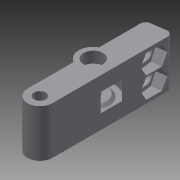
# Autodesk Inventor part: ExtruderSatoerBearingArm
Saved by Autodesk Inventor 2015 SP1 (Build 190203100, 203)
## iProperties
Created: 2015-05-02
Part Number: ExtruderSatoerBearingArm
Material: Generic
Document SubType Name: Modeling
Designer: Jack
Density: 1 g/cm^3
Appearance: Default
Author: Jack
Autodesk Inventor part; units mm, degrees
ref_plane "YZ Plane" through (0, 0, 0) normal (1, 0, 0) x (0, 1, 0)
ref_plane "XZ Plane" through (0, 0, 0) normal (0, 1, 0) x (-1, 0, 0)
ref_plane "XY Plane" through (0, 0, 0) normal (0, 0, 1) x (1, 0, 0)
sketch "Sketch1" plane through (0, 0, 0) normal (0, 0, 1) x (1, 0, 0)
  arc A0 (-4.75, 0) -> (4.75, 0) centre (0, 0) ccw
  line L0 (-4.75, 44.6649) -> (4.75, 46)
  line L1 (4.75, 46) -> (4.75, 0)
  arc A1 (-4.75, 27.0098) -> (-4.75, 17.7902) centre (-1.75, 22.4) ccw
  line L2 (-4.75, 0) -> (-4.75, 17.7902)
  line L3 (-4.75, 27.0098) -> (-4.75, 44.6649)
  dimension "d0" = 9.5
  dimension "d1" = 46
  dimension "d2" = 82
  dimension "d5" = 11
  dimension "d8" = 22.4
  dimension "d9" = 3
  constraints: 8 end point, 4 point on circle, 3 tangent, 3 vertical, 2 centre point, 1 coincident
  measures "d0" diameter of A0
  measures "d1" vertical distance of point (0, 0) L0.end
  measures "d2" angle of L1 L0
  measures "d5" diameter of A1
  measures "d8" vertical distance of point (0, 0) A1.centre
  measures "d9" distance from line of L3 A1.centre
extrude "Extrusion1" add sketch "Sketch1" along normal blind 18
sketch "Sketch4" plane through (0, 0, 18) normal (0, 0, 1) x (1, 0, 0)
  arc A0 (-4.75, 27.0098) -> (-4.75, 17.7902) centre (-1.75, 22.4) ccw projected
sketch "Sketch3" plane through (0, 0, 0) normal (0, 0, -1) x (-1, 0, 0)
  arc A0 (4.75, 17.7902) -> (4.75, 27.0098) centre (1.75, 22.4) ccw projected
  line L0 (1.75, 26.6724) -> (5.45, 24.5362)
  line L1 (5.45, 24.5362) -> (5.45, 20.2638)
  line L2 (5.45, 20.2638) -> (1.75, 18.1276)
  line L3 (1.75, 18.1276) -> (-1.95, 20.2638)
  line L4 (-1.95, 20.2638) -> (-1.95, 24.5362)
  line L5 (-1.95, 24.5362) -> (1.75, 26.6724)
  dimension "d17" = 7.4
  constraints: 12 end point, 1 coincident, 1 vertical, 13 other
  measures "d17" distance between parallel lines of L4 L1
extrude "Extrusion2" [suppressed]
hole "Hole2" at (-1.75, 22.4, 18) direction (0, 0, -1) diameter 4.5 end through all counterbore diameter 7.4 counterbore depth 4.2
ref_plane "Work Plane1" through (0, 0, 9) normal (0, 0, -1) x (-1, 0, 0)
sketch "Sketch5" plane through (0, 0, 9) normal (0, 0, -1) x (-1, 0, 0)
  arc A0 (-4.75, 0) -> (4.75, 0) centre (0, 0) ccw projected
  line L0 (4.75, 17.7902) -> (4.75, 0) projected
  arc A1 (4.75, 17.7902) -> (4.75, 27.0098) centre (1.75, 22.4) ccw projected
  line L1 (4.75, 44.6649) -> (4.75, 27.0098) projected
  line L2 (-4.75, 46) -> (4.75, 44.6649) projected
  line L3 (-4.75, 0) -> (-4.75, 46) projected
  circle A2 centre (1.75, 22.4) radius 8
  dimension "d28" = 16
  constraints: 1 centre point, 1 coincident
  measures "d28" diameter of A2
extrude "Extrusion3" [suppressed]
sketch "Sketch6" plane through (0, 0, 5.5) normal (0, 0, 1) x (1, 0, 0)
  circle A0 centre (-1.75, 22.4) radius 2.25 projected
  circle A1 centre (-1.75, 22.4) radius 5
  point P0 (0, 0)
  dimension "d31" = 10
  constraints: 1 centre point, 1 coincident
  measures "d31" diameter of A1
extrude "Extrusion4" [suppressed]
sketch "Sketch7" plane through (0, 0, 12.5) normal (0, 0, -1) x (-1, 0, 0)
  circle A0 centre (1.75, 22.4) radius 2.25 projected
  circle A1 centre (1.75, 22.4) radius 2.25 projected
  circle A2 centre (1.75, 22.4) radius 5 projected
  point P0 (0, 0)
extrude "Extrusion5" [suppressed]
chamfer "Chamfer1" [suppressed]
fillet "Fillet1" radius 2 2 edges at (-4.75, 44.6649, 9) (4.75, 46, 9)
sketch "Sketch8" plane through (-4.75, 29.8162, 5.5) normal (-1, 0, 0) x (0, 0, 1)
  line L0 (-5.5, 13.1101) -> (-5.5, -2.8064) projected
  line L1 (12.5, 13.1101) -> (12.5, -2.8064) projected
  line L2 (7.5, 7.9636) -> (7.5, 9.5636) construction
  line L3 (9.75, 7.9636) -> (9.75, 9.5636)
  line L4 (5.25, 9.5636) -> (5.25, 7.9636)
  arc A0 (5.25, 7.9636) -> (9.75, 7.9636) centre (7.5, 7.9636) ccw
  arc A1 (9.75, 9.5636) -> (5.25, 9.5636) centre (7.5, 9.5636) ccw
  line L5 (-5.5, 15.8636) -> (12.5, 15.8636) projected
  line L6 (-0.5, 7.9636) -> (-0.5, 9.5636) construction
  line L7 (1.75, 7.9636) -> (1.75, 9.5636)
  line L8 (-2.75, 9.5636) -> (-2.75, 7.9636)
  arc A2 (-2.75, 7.9636) -> (1.75, 7.9636) centre (-0.5, 7.9636) ccw
  arc A3 (1.75, 9.5636) -> (-2.75, 9.5636) centre (-0.5, 9.5636) ccw
  point P0 (-5.5, -29.8162)
  point P1 (7.5, 8.7636)
  point P2 (-0.5, 8.7636)
  dimension "d40" = 1.6
  dimension "d41" = 4.5
  dimension "d42" = 6.3
  dimension "d43" = 5
  dimension "d44" = 5
  constraints: 16 end point, 8 point on circle, 8 tangent, 4 centre point, 3 parallel, 2 midpoint, 2 vertical, 1 equal radius, 1 horizontal alignment
  measures "d40" distance of L2.start L2.end
  measures "d41" diameter of A1
  measures "d42" distance from line of L5 L2.end
  measures "d43" distance from line of L0 point (-0.5, 8.764)
  measures "d44" distance from line of L1 point (7.5, 8.764)
extrude "Extrusion6" cut sketch "Sketch8" against normal up to next
ref_plane "Work Plane2" through (4.75, 43.6993, 0) normal (0.9902681, 0.1391731, 0) x (0, 0, -1)
sketch "Sketch9" plane through (4.75, 43.6993, 0) normal (0.9902681, 0.1391731, 0) x (0, 0, -1)
  ellipse E0 centre (-5, -5.8619) end of major axis (-2.75, -5.8619) minor radius 2.2281 (-7.25, -5.8619) -> (-2.75, -5.8619) ccw projected
  ellipse E1 centre (-5, -4.2774) end of major axis (-7.25, -4.2774) minor radius 2.2281 (-2.75, -4.2774) -> (-7.25, -4.2774) ccw projected
  ellipse E2 centre (-13, -4.2774) end of major axis (-15.25, -4.2774) minor radius 2.2281 (-10.75, -4.2774) -> (-15.25, -4.2774) ccw projected
  ellipse E3 centre (-13, -5.8619) end of major axis (-10.75, -5.8619) minor radius 2.2281 (-15.25, -5.8619) -> (-10.75, -5.8619) ccw projected
  line L0 (-13, -10.1342) -> (-16.7, -7.9981)
  line L1 (-16.7, -7.9981) -> (-16.7, -3.7257)
  line L2 (-16.7, -3.7257) -> (-13, -1.5895)
  line L3 (-13, -1.5895) -> (-9.3, -3.7257)
  line L4 (-9.3, -3.7257) -> (-9.3, -7.9981)
  line L5 (-9.3, -7.9981) -> (-13, -10.1342)
  line L6 (-13, -0.005) -> (-9.3, -2.1412)
  line L7 (-9.3, -2.1412) -> (-9.3, -6.4136)
  line L8 (-9.3, -6.4136) -> (-13, -8.5498)
  line L9 (-13, -8.5498) -> (-16.7, -6.4136)
  line L10 (-16.7, -6.4136) -> (-16.7, -2.1412)
  line L11 (-16.7, -2.1412) -> (-13, -0.005)
  line L12 (-5, -10.1342) -> (-8.7, -7.9981)
  line L13 (-8.7, -7.9981) -> (-8.7, -3.7257)
  line L14 (-8.7, -3.7257) -> (-5, -1.5895)
  line L15 (-5, -1.5895) -> (-1.3, -3.7257)
  line L16 (-1.3, -3.7257) -> (-1.3, -7.9981)
  line L17 (-1.3, -7.9981) -> (-5, -10.1342)
  line L18 (-5, -0.005) -> (-1.3, -2.1412)
  line L19 (-1.3, -2.1412) -> (-1.3, -6.4136)
  line L20 (-1.3, -6.4136) -> (-5, -8.5498)
  line L21 (-5, -8.5498) -> (-8.7, -6.4136)
  line L22 (-8.7, -6.4136) -> (-8.7, -2.1412)
  line L23 (-8.7, -2.1412) -> (-5, -0.005)
  point P0 (0, -42.6129)
  point P1 (-5, -5.8619)
  point P2 (-5, -4.2774)
  dimension "d49" = 7.4
  constraints: 48 end point, 4 coincident, 4 vertical, 3 equal length, 56 other
  measures "d49" distance between parallel lines of L1 L4
extrude "Extrusion7" cut sketch "Sketch9" against normal blind 4
sketch "Sketch10" plane through (0, 0, 0) normal (0, 0, -1) x (-1, 0, 0)
  arc A0 (-4.75, 0) -> (4.75, 0) centre (0, 0) ccw projected
hole "Hole3" at (0, 0, 0) direction (0, 0, 1) diameter 4.5 end through all
body "Solid1"
